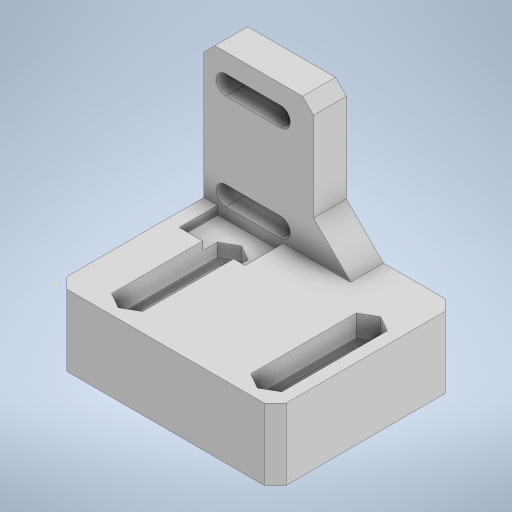
# Autodesk Inventor part: Motor Mount
Saved by Autodesk Inventor 2024 (Build 280153020, 153B)
## iProperties
Created: 2024-02-12
Part Number: Motor Mount
Material: Generic
Document SubType Name: Modeling
Designer: scottst
Density: 1 g/cm^3
Appearance: Default
Author: scottst
Autodesk Inventor part; units mm, degrees
ref_plane "YZ Plane" through (0, 0, 0) normal (1, 0, 0) x (0, 1, 0)
ref_plane "XZ Plane" through (0, 0, 0) normal (0, 1, 0) x (-1, 0, 0)
ref_plane "XY Plane" through (0, 0, 0) normal (0, 0, 1) x (1, 0, 0)
sketch "Sketch1" plane through (0, 0, 0) normal (1, 0, 0) x (0, 1, 0)
  line L0 (0, 0) -> (13, 0)
  line L1 (13, 0) -> (13, -27)
  line L2 (13, -27) -> (0, -27)
  line L3 (0, -27) -> (0, 0)
  dimension "d0" = 13
  dimension "d1" = 27
  constraints: 8 end point, 2 parallel, 1 horizontal, 1 perpendicular
  measures "d0" distance of L1.end L2.end
  measures "d1" distance of L0.end L1.end
extrude "Extrusion1" add sketch "Sketch1" along normal blind 40
sketch "Sketch2" plane through (40, 0, 0) normal (1, 0, 0) x (0, 0, -1)
  line L0 (27, 0) -> (27, 13) projected
  line L1 (27, 0) -> (33, 0)
  line L2 (33, 0) -> (33, 38)
  line L3 (33, 38) -> (27, 38)
  line L4 (27, 38) -> (27, 0)
  point P0 (0, 0)
  dimension "d4" = 6
  dimension "d5" = 38
  constraints: 8 end point, 2 parallel, 1 horizontal, 1 perpendicular
  measures "d4" distance of L3.end L2.end
  measures "d5" distance of L2.end L1.end
extrude "Extrusion2" add sketch "Sketch2" against normal blind 40
sketch "Sketch3" plane through (0, 13, 0) normal (0, 1, 0) x (1, 0, 0)
  line L0 (40, 27) -> (40, 0) construction
  line L1 (40, 0) -> (35, 0) construction
  line L2 (0, 0) -> (40, 0) construction
  line L3 (35, 0) -> (35, 5) construction
  line L4 (35, 5) -> (35, 21) construction
  line L5 (35, 5) -> (9.6, 5) construction
  line L6 (35, 5) -> (35, 21) construction
  line L7 (36.65, 5) -> (36.65, 21)
  line L8 (33.35, 21) -> (33.35, 5)
  arc A0 (33.35, 5) -> (36.65, 5) centre (35, 5) ccw
  arc A1 (36.65, 21) -> (33.35, 21) centre (35, 21) ccw
  line L9 (9.6, 0) -> (9.6, 5) construction
  line L10 (9.6, 5) -> (9.6, 21) construction
  line L11 (9.6, 5) -> (-15.8, 5) construction
  line L12 (9.6, 5) -> (9.6, 21) construction
  line L13 (11.25, 5) -> (11.25, 21)
  line L14 (7.95, 21) -> (7.95, 5)
  arc A2 (7.95, 5) -> (11.25, 5) centre (9.6, 5) ccw
  arc A3 (11.25, 21) -> (7.95, 21) centre (9.6, 21) ccw
  point P0 (35, 13)
  point P1 (9.6, 13)
  dimension "d8" = 5
  dimension "d9" = 5
  dimension "d10" = 16
  dimension "d11" = 25.4
  dimension "d12" = 3.3
  dimension "d13" = 5
  dimension "d14" = 16
  dimension "d15" = 25.4
  dimension "d16" = 3.3
  constraints: 30 end point, 8 point on circle, 8 tangent, 4 centre point, 4 equal length, 3 point on line, 2 horizontal, 2 midpoint, 1 perpendicular
  measures "d8" distance of L0.end L1.end
  measures "d9" distance of L1.end L3.end
  measures "d10" distance of L3.end L4.end
  measures "d11" distance of L3.end L5.end
  measures "d12" diameter of A1
  measures "d13" distance of L9.start L9.end
  measures "d14" distance of L9.end L10.end
  measures "d15" distance of L9.end L11.end
  measures "d16" diameter of A3
extrude "Extrusion3" cut sketch "Sketch3" against normal blind 40
sketch "Sketch4" plane through (0, 13, 0) normal (0, 1, 0) x (1, 0, 0)
  point P0 (0, 0)
sketch "Sketch5" plane through (0, 13, 0) normal (0, 1, 0) x (1, 0, 0)
  arc A0 (33.35, 5) -> (36.65, 5) centre (35, 5) ccw projected
  line L0 (35, 5) -> (32.1806, 5) construction
  line L1 (35, 5) -> (37.8194, 5) construction
  line L2 (37.8194, 6.6278) -> (37.8194, 3.3722)
  line L3 (37.8194, 3.3722) -> (35, 1.7444)
  line L4 (35, 1.7444) -> (32.1806, 3.3722)
  line L5 (32.1806, 3.3722) -> (32.1806, 6.6278)
  arc A1 (36.65, 21) -> (33.35, 21) centre (35, 21) ccw projected
  line L6 (35, 21) -> (32.1806, 21) construction
  line L7 (32.1806, 22.6278) -> (35, 24.2556)
  line L8 (35, 24.2556) -> (37.8194, 22.6278)
  line L9 (37.8194, 22.6278) -> (37.8194, 19.3722)
  line L10 (32.1806, 19.3722) -> (32.1806, 22.6278)
  line L11 (32.1806, 19.3722) -> (32.1806, 6.6278)
  line L12 (33.35, 5) -> (33.35, 21) projected
  line L13 (36.65, 5) -> (36.65, 21) projected
  line L14 (37.8194, 19.3722) -> (37.8194, 6.6278)
  arc A2 (7.95, 5) -> (11.25, 5) centre (9.6, 5) ccw projected
  line L15 (9.6, 5) -> (6.7806, 5) construction
  line L16 (9.6, 5) -> (12.4194, 5) construction
  line L17 (12.4194, 6.6278) -> (12.4194, 3.3722)
  line L18 (12.4194, 3.3722) -> (9.6, 1.7444)
  line L19 (9.6, 1.7444) -> (6.7806, 3.3722)
  line L20 (6.7806, 3.3722) -> (6.7806, 6.6278)
  line L21 (9.6, 21) -> (6.7806, 21) construction
  line L22 (6.7806, 22.6278) -> (9.6, 24.2556)
  line L23 (9.6, 24.2556) -> (12.4194, 22.6278)
  line L24 (12.4194, 22.6278) -> (12.4194, 19.3722)
  line L25 (6.7806, 19.3722) -> (6.7806, 22.6278)
  line L26 (6.7806, 19.3722) -> (6.7806, 6.6278)
  line L27 (12.4194, 19.3722) -> (12.4194, 6.6278)
  point P0 (0, 0)
  dimension "d19" = 2.8194
  dimension "d20" = 2.8194
  dimension "d21" = 2.8194
  dimension "d23" = 2.8194
  dimension "d24" = 2.8194
  dimension "d25" = 2.8194
  constraints: 52 end point, 6 horizontal, 4 coincident, 4 midpoint, 1 parallel, 32 other
  measures "d19" distance of L0.start L0.end
  measures "d20" distance of L0.start L1.end
  measures "d21" distance of L6.start L6.end
  measures "d23" distance of L15.start L15.end
  measures "d24" distance of L15.start L16.end
  measures "d25" distance of L21.start L21.end
extrude "Extrusion4" cut sketch "Sketch5" against normal blind 4 contours L12 A1 L13 A0 | L2 L3 L4 L5 L11 L10 L7 L8 L9 L14 | L17 L18 L19 L20 L26 L25 L22 L23 L24 L27
sketch "Sketch6" plane through (40, 13, -27) normal (0, 0, 1) x (1, 0, 0)
  line L0 (-40, 0) -> (0, 0) construction
  line L1 (-40, 0) -> (-40, 2.3) construction
  line L2 (-40, 25) -> (-40, -13) construction
  line L3 (-40, 2.3) -> (-6.5941, 2.3) construction
  line L4 (-40, 2.3) -> (-40, 19.8) construction
  line L5 (-40, 19.8) -> (-7.5372, 19.8) construction
  line L6 (-40, 2.3) -> (-36, 2.3) construction
  line L7 (-36, 2.3) -> (-36, 19.8) construction
  line L8 (-36, 19.8) -> (-26, 19.8) construction
  line L9 (-36, 2.3) -> (-26, 2.3) construction
  line L10 (-36, 19.8) -> (-26, 19.8) construction
  line L11 (-36, 18.05) -> (-26, 18.05)
  line L12 (-26, 21.55) -> (-36, 21.55)
  arc A0 (-36, 21.55) -> (-36, 18.05) centre (-36, 19.8) ccw
  arc A1 (-26, 18.05) -> (-26, 21.55) centre (-26, 19.8) ccw
  line L13 (-36, 2.3) -> (-26, 2.3) construction
  line L14 (-36, 0.55) -> (-26, 0.55)
  line L15 (-26, 4.05) -> (-36, 4.05)
  arc A2 (-36, 4.05) -> (-36, 0.55) centre (-36, 2.3) ccw
  arc A3 (-26, 0.55) -> (-26, 4.05) centre (-26, 2.3) ccw
  point P0 (-31, 19.8)
  point P1 (-31, 2.3)
  dimension "d28" = 2.3
  dimension "d29" = 17.5
  dimension "d30" = 4
  dimension "d31" = 10
  dimension "d32" = 10
  dimension "d33" = 3.5
  dimension "d34" = 3.5
  constraints: 32 end point, 8 point on circle, 8 tangent, 6 point on line, 4 centre point, 3 perpendicular, 2 collinear, 2 midpoint, 2 parallel
  measures "d28" distance of L0.start L1.end
  measures "d29" distance of L1.end L4.end
  measures "d30" distance of L1.end L6.end
  measures "d31" distance of L7.end L8.end
  measures "d32" distance of L6.end L9.end
  measures "d33" diameter of A1
  measures "d34" diameter of A3
extrude "Extrusion5" cut sketch "Sketch6" against normal blind 35.6875
sketch "Sketch7" plane through (40, 13, -27) normal (0, 0, 1) x (1, 0, 0)
  line L0 (0, 25) -> (0, 0) projected
  line L1 (-40, 0) -> (0, 0) projected
  line L2 (0, 25) -> (-20, 25)
  line L3 (-20, 25) -> (-20, 0)
  line L4 (-20, 0) -> (0, 0)
  line L5 (0, 0) -> (0, 25)
  point P0 (-40, -13)
  constraints: 8 end point, 2 parallel, 1 horizontal, 1 midpoint, 1 perpendicular
extrude "Extrusion6" cut sketch "Sketch7" against normal blind 45.275
chamfer "Chamfer1" distance 6.7625 angle 45 1 edges at (20, 13, -30)
chamfer "Chamfer2" distance 2 angle 45 1 edges at (20, 38, -30)
chamfer "Chamfer3" distance 2 angle 45 1 edges at (0, 38, -30)
chamfer "Chamfer4" distance 2 angle 45 4 edges at (40, 6.5, 0) (0, 6.5, 0) (40, 6.5, -33) (0, 18, -33)
sketch "Sketch8" plane through (0, 13, -27) normal (0, 1, 0) x (1, 0, 0)
  line L0 (0, 0) -> (26.7625, 0) construction
  line L1 (0, 0) -> (2.5, 0) construction
  line L2 (2.5, 0) -> (14.5, 0)
  line L3 (14.5, 0) -> (14.5, -7)
  line L4 (14.5, -7) -> (2.5, -7)
  line L5 (2.5, -7) -> (2.5, 0)
  point P0 (0, -27)
  dimension "d53" = 2.5
  dimension "d54" = 12
  dimension "d55" = 7
  constraints: 10 end point, 2 parallel, 1 horizontal, 1 perpendicular, 1 point on line
  measures "d53" distance of L0.start L1.end
  measures "d54" distance of L3.end L4.end
  measures "d55" distance of L2.end L3.end
extrude "Extrusion7" cut sketch "Sketch8" against normal blind 1.5
body "Solid1"
